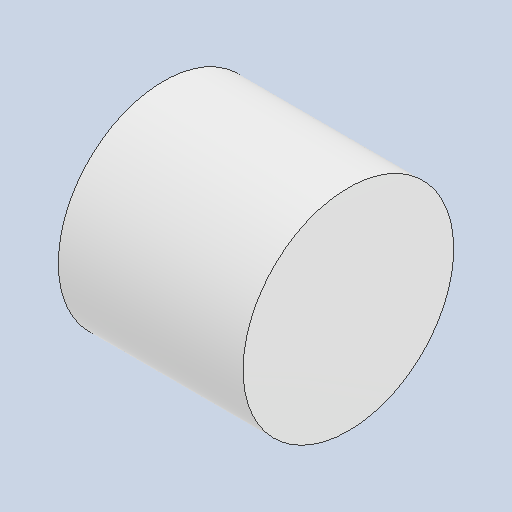
# Autodesk Inventor part: AnpresspinnAufnahme_Buchse
Saved by Autodesk Inventor 2024 (Build 280153000, 153)
## iProperties
Created: 2022-08-21
Part Number: AnpresspinnAufnahme_Buchse
Material: PBT-Kunststoff
Document SubType Name: Modeling
Designer: alexw
Density: 1.31 g/cm^3
Appearance: Glatt - Weiß
Mass: 0.148158 g
Surface Area: 1.88496 cm^2
Volume: 0.113097 cm^3
Author: alexw
Autodesk Inventor part; units mm, degrees
ref_plane "YZ Plane" through (0, 0, 0) normal (1, 0, 0) x (0, 1, 0)
ref_plane "XZ Plane" through (0, 0, 0) normal (0, 1, 0) x (-1, 0, 0)
ref_plane "XY Plane" through (0, 0, 0) normal (0, 0, 1) x (1, 0, 0)
sketch "Skizze1" plane through (0, 0, 0) normal (0, 0, 1) x (1, 0, 0)
  line L0 (4, 0) -> (4, 1.5)
  line L1 (4, 1.5) -> (0, 1.5)
  line L2 (0, 1.5) -> (0, 3)
  line L3 (0, 3) -> (5, 3)
  line L4 (5, 3) -> (5, 0)
  line L5 (9, 0) -> (4, 0)
  line L6 (0, 0) -> (5, 0) construction
  line L7 (0, -0.6) -> (0, 3.6) construction
  point P0 (5, 0)
  dimension "d0" = 3
  dimension "d2" = 6
  dimension "d4" = 4
  dimension "d5" = 5
  constraints: 15 end point, 4 perpendicular, 2 collinear, 1 horizontal, 1 vertical
  measures "d0" diameter of L1 L6
  measures "d2" diameter of L3 L6
  measures "d4" distance between parallel lines of L0 L7
  measures "d5" distance between parallel lines of L4 L2
revolve "Umdrehung1" add sketch "Skizze1" angle 360 about axis through (0, 0, 0) along (1, 0, 0)
thicken "Thicken1" operation add thickness 0.15 both sides no extend neighbours yes toward (0, -0.9967573, 0.0804666) faces at (1.6667, 2.9903, -0.2414)
